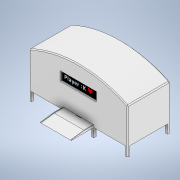
# Autodesk Inventor part: Twist Body
Saved by Autodesk Inventor 2021 (Build 250183000, 183)
## iProperties
Created: 2021-03-24
Part Number: Twist Body
Material: Generic
Document SubType Name: Modeling
Designer: calst
Density: 1 g/cm^3
Appearance: Smooth - White
Author: calst
Autodesk Inventor part; units mm, degrees
ref_plane "YZ Plane" through (0, 0, 0) normal (1, 0, 0) x (0, 1, 0)
ref_plane "XZ Plane" through (0, 0, 0) normal (0, 1, 0) x (-1, 0, 0)
ref_plane "XY Plane" through (0, 0, 0) normal (0, 0, 1) x (1, 0, 0)
sketch "Sketch1" plane through (0, 0, 0) normal (0, 1, 0) x (-1, 0, 0)
  line L0 (0, 0) -> (68.5, 0)
  line L1 (68.5, 0) -> (68.5, -94)
  line L2 (68.5, -94) -> (0, -94)
  line L3 (0, -94) -> (0, 0)
  dimension "d0" = 94
  dimension "d1" = 68.5
  constraints: 8 end point, 2 parallel, 1 horizontal, 1 perpendicular
  measures "d0" distance of L0.end L1.end
  measures "d1" distance of L1.end L2.end
extrude "Extrusion1" add sketch "Sketch1" along normal blind 4
sketch "Sketch2" plane through (0, 4, 0) normal (0, 1, 0) x (1, 0, 0)
  line L0 (0, 94) -> (-68.5, 94) projected
  line L1 (-68.5, 0) -> (0, 0) projected
  line L2 (-34.25, 0) -> (-39.25, 0)
  line L3 (-39.25, 0) -> (-39.25, 94)
  line L4 (-39.25, 94) -> (-29.25, 94)
  line L5 (-29.25, 94) -> (-29.25, 0)
  line L6 (-29.25, 0) -> (-34.25, 0)
  point P0 (-29.25, 0)
  dimension "d4" = 5
  dimension "d5" = 10
  constraints: 10 end point, 4 perpendicular, 1 midpoint, 1 point on line
  measures "d4" distance of L2.start L2.end
  measures "d5" distance of L3.end L4.end
extrude "Extrusion2" cut sketch "Sketch2" against normal blind 5
sketch "Sketch3" plane through (0, 4, 0) normal (0, 1, 0) x (1, 0, 0)
  line L0 (-39.25, 94) -> (-68.5, 94) projected
  line L1 (-68.5, 94) -> (-64.1699, 94)
  line L2 (-66, 89) -> (-68.5, 89)
  line L3 (-68.5, 89) -> (-68.5, 94)
  line L4 (-66, 89) -> (-66, 91.5)
  line L5 (-66, 91.5) -> (-64.1699, 91.5)
  line L6 (-64.1699, 94) -> (-68.5, 94)
  line L7 (-68.5, 94) -> (-68.5, 0) projected
  line L8 (-68.5, 89) -> (-68.5, 94)
  line L9 (0, 94) -> (-5, 94)
  line L10 (0, 94) -> (-29.25, 94) projected
  line L11 (-5, 91.5) -> (-2.5, 91.5)
  line L12 (-2.5, 91.5) -> (-2.5, 89)
  line L13 (0, 0) -> (0, 94) projected
  line L14 (0, 89) -> (0, 94)
  line L15 (-64.1699, 91.5) -> (-5, 91.5)
  line L16 (-64.1699, 94) -> (-5, 94)
  line L17 (0, 89) -> (0, 0)
  line L18 (0, 0) -> (-68.5, 0)
  line L19 (-68.5, 0) -> (-68.5, 89)
  line L20 (-66, 89) -> (-66, 2.5)
  line L21 (-68.5, 0) -> (-39.25, 0) projected
  line L22 (-66, 2.5) -> (-2.5, 2.5)
  line L23 (-2.5, 2.5) -> (-2.5, 89)
  dimension "d8" = 5
  dimension "d9" = 5
  dimension "d11" = 2.5
  dimension "d12" = 2.5
  dimension "d13" = 2.5
  dimension "d15" = 86.5
  constraints: 38 end point, 5 perpendicular, 4 collinear, 2 horizontal, 2 parallel, 1 point on line, 1 vertical
  measures "d8" distance of L5.end L2.end
  measures "d9" distance of L2.end L0.end
  measures "d11" distance of L9.end L11.start
  measures "d12" distance of L1.end L5.end
  measures "d13" distance of L2.start L4.end
  measures "d15" distance of L2.start L20.end
extrude "Extrusion3" add sketch "Sketch3" along normal blind 5
sketch "Sketch4" plane through (-29.25, 0, 0) normal (0, 0, 1) x (1, 0, 0)
  line L0 (-10, 4) -> (-36.75, 4) projected
  line L1 (26.75, 4) -> (0, 4) projected
  line L2 (-36.75, 4) -> (26.75, 4)
  line L3 (26.75, 4) -> (26.75, 5.1)
  line L4 (-36.75, 4) -> (-36.75, 5.1)
  line L5 (-36.75, 5.1) -> (26.75, 5.1)
  point P0 (29.25, 0)
  point P1 (-39.25, 9)
  dimension "d19" = 1.1
  dimension "d20" = 1.1
  constraints: 8 end point, 2 perpendicular, 1 collinear
  measures "d19" distance of L1.start L3.end
  measures "d20" distance of L0.end L4.end
extrude "Extrusion4" cut sketch "Sketch4" against normal blind 5
sketch "Sketch5" plane through (0, 9, 0) normal (0, 1, 0) x (1, 0, 0)
  line L0 (-66, 2.5) -> (-66, 91.5) projected
  line L1 (-68.5, 94) -> (-68.5, 0) projected
  line L2 (-66, 91.5) -> (-68.5, 91.5)
  line L3 (-68.5, 91.5) -> (-68.5, 94)
  line L4 (-68.5, 94) -> (-66, 94)
  line L5 (-66, 94) -> (-66, 91.5)
  line L6 (0, 0) -> (0, 94) projected
  line L7 (-2.5, 91.5) -> (-29.25, 91.5) projected
  line L8 (0, 94) -> (-2.5, 94)
  line L9 (-2.5, 94) -> (-2.5, 91.5)
  line L10 (-2.5, 91.5) -> (0, 91.5)
  line L11 (0, 91.5) -> (0, 94)
  line L12 (-68.5, 0.034) -> (-66, 0.034)
  line L13 (-66, 0.034) -> (-66, 2.534)
  line L14 (-66, 2.534) -> (-68.5, 2.534)
  line L15 (-68.5, 2.534) -> (-68.5, 0.034)
  line L16 (-2.5, 2.5) -> (-66, 2.5) projected
  line L17 (-68.5, 0) -> (0, 0) projected
  line L18 (-2.5, 2.5) -> (0, 2.5)
  line L19 (0, 2.5) -> (0, 0)
  line L20 (0, 0) -> (-2.5, 0)
  line L21 (-2.5, 0) -> (-2.5, 2.5)
  dimension "d23" = 2.5
  constraints: 32 end point, 8 parallel, 4 horizontal, 4 perpendicular, 2 point on line, 1 other
  measures "d23" distance of L12.end L13.end
extrude "Extrusion5" add sketch "Sketch5" along normal blind 30 contours L13 L12 L1 L14 L0 | L18 L6 L17 L21 | L2 L1 L4 L5 | L10 L9 L8 L6
sketch "Sketch6" plane through (0, 4, 0) normal (0, 1, 0) x (1, 0, 0)
  line L0 (-39.25, 94) -> (-68.5, 94) projected
  line L1 (-68.5, 94) -> (-66.2, 94)
  line L2 (-66.2, 94) -> (-66.2, 91.7)
  line L3 (-68.5, 91.5) -> (-66, 91.5) projected
  line L4 (0, 0) -> (0, 94) projected
  line L5 (0, 0) -> (-2.3, 0)
  line L6 (-29.25, 0) -> (0, 0) projected
  line L7 (-2.3, 0) -> (-2.3, 2.3)
  line L8 (-66.2, 91.7) -> (-2.3, 91.7)
  line L9 (-2.3, 91.7) -> (-2.3, 2.3)
  line L10 (-2.3, 2.3) -> (-66.2, 2.3)
  line L11 (-66.2, 2.3) -> (-66.2, 91.7)
  dimension "d26" = 2.3
  dimension "d27" = 2.3
  dimension "d28" = 2.3
  dimension "d29" = 2.3
  constraints: 16 end point, 3 perpendicular, 2 parallel, 2 point on line, 1 horizontal
  measures "d26" distance of L0.end L1.end
  measures "d27" distance of L1.end L2.end
  measures "d28" distance of L4.start L5.end
  measures "d29" distance of L5.end L7.end
extrude "Extrusion6" cut sketch "Sketch6" along normal blind 50
sketch "Sketch8" plane through (0, 0, 0) normal (1, 0, 0) x (0, 0, -1)
  line L0 (0, 4) -> (91.7, 4) projected
  line L1 (0, 4) -> (-20, 4)
  line L2 (-50, 0) -> (-20, 4)
  line L3 (0, 4) -> (0, 0) projected
  line L4 (-50, 0) -> (0, 0)
  dimension "d32" = 20
  constraints: 6 end point, 1 collinear, 1 horizontal
  measures "d32" distance of L0.start L1.end
extrude "Extrusion7" add sketch "Sketch8" against normal blind 68.5
sketch "Sketch10" plane through (0, 0, -94) normal (1, 0, 0) x (0, 0, -1)
  line L0 (-114, 4) -> (-94, 4) projected
  line L1 (-94, 5.1) -> (-91.7, 5.1) projected
  line L2 (-114, 5.1) -> (-94, 5.1)
  line L3 (-114, 4) -> (-144, 0) projected
  line L4 (-144, 0) -> (-144, 1.1)
  line L5 (-144, 1.1) -> (-114, 5.1)
  line L6 (-144, 0) -> (-114, 4)
  line L7 (-94, 4) -> (-94, 5.1)
  line L8 (-94, 4) -> (-91.7, 4) projected
  line L9 (-94, 4) -> (-114, 4)
  point P0 (-94, 0)
  dimension "d37" = 1.1
  constraints: 12 end point, 1 collinear, 1 perpendicular, 1 vertical
  measures "d37" distance of L3.end L4.end
extrude "Extrusion8" add sketch "Sketch10" against normal blind 1
sketch "Sketch11" plane through (-68.5, 4, 0) normal (-1, 0, 0) x (0, 0, 1)
  line L0 (50, -4) -> (20, 0) projected
  line L1 (50, -4) -> (50, -2.9) projected
  line L2 (50, -4) -> (50, -2.9)
  line L3 (20, 1.1) -> (0, 1.1) projected
  line L4 (50, -2.9) -> (20, 1.1)
  line L5 (20, 1.1) -> (0, 1.1)
  line L6 (0, 1.1) -> (0, 0) projected
  line L7 (0, 1.1) -> (0, 0)
  line L8 (20, 0) -> (0, 0) projected
  line L9 (0, 0) -> (20, 0)
  line L10 (50, -4) -> (-94, -4) projected
  line L11 (20, 0) -> (50, -4)
  point P0 (0, -4)
  constraints: 12 end point, 4 equal length, 1 perpendicular
extrude "Extrusion9" add sketch "Sketch11" against normal blind 1
sketch "Sketch15" plane through (-66.2, 4, -91.7) normal (0, 0, 1) x (1, 0, 0)
  line L0 (26.95, 0) -> (36.95, 0)
  line L1 (36.95, 0) -> (36.95, 1.1)
  line L2 (36.95, 1.1) -> (26.95, 1.1)
  line L3 (26.95, 1.1) -> (26.95, 0)
  point P0 (66.2, -4)
  dimension "d56" = 1.1
  constraints: 8 end point, 2 parallel, 1 horizontal, 1 perpendicular
  measures "d56" distance of L0.end L1.end
extrude "Extrusion13" cut sketch "Sketch15" against normal blind 94
sketch "Sketch17" plane through (0, 0, 0) normal (0, -1, 0) x (1, 0, 0)
  line L0 (-29.25, -81.7) -> (-24.25, -81.7)
  line L1 (-24.25, -81.7) -> (-24.25, -101.7)
  line L2 (-24.25, -101.7) -> (-29.25, -101.7)
  line L3 (-29.25, -101.7) -> (-29.25, -81.7)
  line L4 (-66, -2.3) -> (-2.5, -2.3) projected
  line L5 (-29.25, 0) -> (-39.25, 0) projected
  line L6 (-2.5, -2.3) -> (-66, -2.3) projected
  line L7 (-29.25, -2.3) -> (-29.25, -12.3)
  line L8 (-29.25, -91.7) -> (-29.25, 0) projected
  line L9 (-29.25, -12.3) -> (-24.25, -12.3)
  line L10 (-24.25, -12.3) -> (-24.25, 7.7)
  line L11 (-24.25, 7.7) -> (-29.25, 7.7)
  line L12 (-29.25, 7.7) -> (-29.25, -2.3)
  line L13 (-39.25, -2.3) -> (-39.25, -12.3)
  line L14 (-39.25, 0) -> (-39.25, -91.7) projected
  line L15 (-39.25, -12.3) -> (-44.25, -12.3)
  line L16 (-44.25, -12.3) -> (-44.25, 7.7)
  line L17 (-44.25, 7.7) -> (-39.25, 7.7)
  line L18 (-39.25, 7.7) -> (-39.25, -2.3)
  point P0 (0, 0)
  point P1 (-39.25, -81.7)
  dimension "d76" = 2.3
  dimension "d77" = 10
  dimension "d78" = 5
  dimension "d79" = 20
  constraints: 28 end point, 7 perpendicular, 6 point on line, 2 collinear, 1 horizontal
  measures "d76" distance between parallel lines of L4 L5
  measures "d77" distance of L7.start L7.end
  measures "d78" distance of L7.end L9.end
  measures "d79" distance of L9.end L10.end
extrude "Extrusion14" add sketch "Sketch17" along normal blind 20 contours L0 L1 L2 L3 | L13 L15 L16 L4 | L4 L16 L17 L18 L14 | L8 L12 L11 L10 L4 | L4 L10 L9 L7
fillet "Fillet1" radius 10 6 edges at (-26.75, -20, -81.7) (-26.75, -20, -101.7) (-26.75, -20, 7.7) (-26.75, -20, -12.3) (-41.75, -20, -12.3) (-41.75, -20, 7.7)
sketch "Sketch19" plane through (-24.25, 0, 7.7) normal (1, 0, 0) x (0, 0, -1)
  arc A0 (0, -10) -> (20, -10) centre (10, -10) ccw projected
  circle A1 centre (10, -10) radius 2.5
  arc A2 (89.4, -10) -> (109.4, -10) centre (99.4, -10) ccw projected
  circle A3 centre (99.4, -10) radius 2.5
  point P0 (7.7, 0)
  dimension "d80" = 5
  dimension "d81" = 5
  constraints: 2 centre point, 2 coincident
  measures "d80" diameter of A1
  measures "d81" diameter of A3
extrude "Extrusion16" cut sketch "Sketch19" against normal blind 30
sketch "Sketch21" plane through (0, 0, 0) normal (0, -1, 0) x (1, 0, 0)
  line L0 (-68.5, -94) -> (-63.5, -94)
  line L1 (-63.5, -94) -> (-63.5, -89)
  line L2 (-63.5, -89) -> (-68.5, -89)
  line L3 (-68.5, -89) -> (-68.5, -94)
  line L4 (-67.5, 50) -> (-68.5, 50) projected
  line L5 (0, 50) -> (-1, 50) projected
  line L6 (0, -94) -> (-2.5, -94) projected
  line L7 (0, -94) -> (-5, -94)
  line L8 (-5, -94) -> (-5, -89)
  line L9 (-5, -89) -> (0, -89)
  line L10 (0, -89) -> (0, -94)
  dimension "d84" = 5
  dimension "d85" = 5
  constraints: 16 end point, 4 parallel, 2 horizontal, 2 perpendicular
  measures "d84" distance of L0.end L1.end
  measures "d85" distance of L1.end L2.end
extrude "Extrusion17" add sketch "Sketch21" along normal blind 20
sketch "Sketch23" plane through (0, 9, -91.5) normal (1, 0, 0) x (0, 0, -1)
  point P0 (-91.5, -9)
sketch "Sketch24" plane through (0, 0, 0) normal (0, -1, 0) x (1, 0, 0)
  line L0 (0, 0) -> (-5, 0)
  line L1 (-5, 0) -> (-5, -5)
  line L2 (-5, -5) -> (0, -5)
  line L3 (0, -5) -> (0, 0)
  line L4 (-68.5, -0.034) -> (-68.5, 0) projected
  line L5 (-68.5, 0) -> (-63.5, 0)
  line L6 (-63.5, 0) -> (-63.5, -5)
  line L7 (-63.5, -5) -> (-68.5, -5)
  line L8 (-68.5, -5) -> (-68.5, 0)
  dimension "d94" = 5
  dimension "d95" = 5
  dimension "d96" = 5
  constraints: 16 end point, 4 parallel, 2 horizontal, 2 perpendicular
  measures "d94" distance of L2.end L1.end
  measures "d95" distance of L0.end L1.end
  measures "d96" distance of L6.end L7.end
extrude "Extrusion18" add sketch "Sketch24" along normal blind 20
sketch "Sketch25" plane through (0, 9, -91.5) normal (1, 0, 0) x (0, 0, -1)
  line L0 (-91.466, 0) -> (-91.5, 0) projected
  line L1 (-9.8, -9) -> (2.5, -9) projected
  line L2 (-91.5, 0) -> (2.5, 0)
  line L3 (2.5, 0) -> (2.5, -9)
  line L4 (2.5, -9) -> (-91.5, -9)
  line L5 (-91.5, -9) -> (-91.5, 0)
  point P0 (-91.5, -9)
  constraints: 8 end point, 2 parallel, 1 horizontal, 1 perpendicular
extrude "Extrusion19" add sketch "Sketch25" along normal blind 75
sketch "Sketch26" plane through (-68.5, 9, -0.034) normal (-1, 0, 0) x (0, 0, 1)
  line L0 (0.034, -9) -> (0.034, -29) projected
  line L1 (-93.966, 0) -> (0.034, 0)
  line L2 (0.034, 0) -> (0.034, -9)
  line L3 (0.034, -9) -> (-93.966, -9)
  line L4 (-93.966, -9) -> (-93.966, 0)
  constraints: 8 end point, 2 parallel, 1 horizontal, 1 perpendicular
extrude "Extrusion20" add sketch "Sketch26" along normal blind 75
sketch "Sketch28" plane through (0, 0, 0) normal (0, -1, 0) x (1, 0, 0)
  line L0 (-68.5, -94) -> (-143.5, -94) projected
  line L1 (-143.5, -94) -> (-138.5, -94)
  line L2 (-138.5, -94) -> (-138.5, -89)
  line L3 (-138.5, -89) -> (-143.5, -89)
  line L4 (-143.5, -89) -> (-143.5, -94)
  line L5 (-143.5, -94) -> (-143.5, 0) projected
  line L6 (-143.5, 0) -> (-138.5, 0)
  line L7 (-138.5, 0) -> (-138.5, -5)
  line L8 (-138.5, -5) -> (-143.5, -5)
  line L9 (-143.5, -5) -> (-143.5, 0)
  line L10 (0, -94) -> (75, -94) projected
  line L11 (75, -94) -> (70, -94)
  line L12 (70, -94) -> (70, -89)
  line L13 (70, -89) -> (75, -89)
  line L14 (75, -89) -> (75, -94)
  line L15 (75, -94) -> (75, 0) projected
  line L16 (75, 0) -> (70, 0)
  line L17 (70, 0) -> (70, -5)
  line L18 (70, -5) -> (75, -5)
  line L19 (75, -5) -> (75, 0)
  point P0 (0, 0)
  dimension "d103" = 5
  dimension "d104" = 5
  dimension "d105" = 5
  dimension "d106" = 5
  dimension "d107" = 5
  dimension "d108" = 5
  constraints: 32 end point, 8 parallel, 4 horizontal, 4 perpendicular, 2 point on line
  measures "d103" distance of L3.end L2.end
  measures "d104" distance of L12.end L13.end
  measures "d105" distance of L18.end L17.end
  measures "d106" distance of L6.end L7.end
  measures "d107" distance of L1.end L2.end
  measures "d108" distance of L16.end L17.end
extrude "Extrusion21" add sketch "Sketch28" along normal blind 20
sketch "Sketch29" plane through (0, 9, 0) normal (0, 1, 0) x (1, 0, 0)
  point P0 (0, 0)
sketch "Sketch30" plane through (0, 9, 0) normal (0, 1, 0) x (1, 0, 0)
  line L0 (2.7, 89) -> (70, 89)
  line L1 (70, 89) -> (70, 5)
  line L2 (70, 5) -> (2.7, 5)
  line L3 (2.7, 5) -> (2.7, 89)
  line L4 (-138.5, 94) -> (-138.5, 89) projected
  line L5 (-138.5, 89) -> (-71.2, 89)
  line L6 (-71.2, 89) -> (-71.2, 5)
  line L7 (-71.2, 5) -> (-138.5, 5)
  line L8 (-138.5, 5) -> (-138.5, 89)
  line L9 (-2.5, 0) -> (-143.5, 0) projected
  line L10 (-66.2, 2.534) -> (-66.2, 91.5) projected
  line L11 (0, 94) -> (75, 94) projected
  line L12 (75, 94) -> (75, 0) projected
  line L13 (-2.3, 91.5) -> (-2.3, 2.5) projected
  point P0 (0, 0)
  dimension "d111" = 5
  dimension "d112" = 5
  dimension "d113" = 5
  dimension "d114" = 5
  dimension "d115" = 5
  constraints: 16 end point, 4 parallel, 2 horizontal, 2 perpendicular, 1 point on line
  measures "d111" distance between parallel lines of L9 L7
  measures "d112" distance between parallel lines of L10 L6
  measures "d113" distance between parallel lines of L11 L0
  measures "d114" distance between parallel lines of L12 L1
  measures "d115" distance between parallel lines of L13 L3
extrude "Extrusion22" cut sketch "Sketch30" against normal blind 5
sketch "Sketch32" plane through (0, 9, 0) normal (0, 1, 0) x (1, 0, 0)
  line L0 (-68.5, 94) -> (-143.5, 94) projected
  line L1 (75, 5) -> (75, 0) projected
  line L2 (-143.5, 94) -> (75, 94)
  line L3 (75, 94) -> (75, 0)
  line L4 (75, 0) -> (-143.5, 0)
  line L5 (-143.5, 0) -> (-143.5, 94)
  line L6 (-71.2, 89) -> (-71.2, 5) projected
  line L7 (-138.5, 89) -> (-71.2, 89)
  line L8 (-71.2, 89) -> (-71.2, 5)
  line L9 (-71.2, 5) -> (-138.5, 5)
  line L10 (-138.5, 5) -> (-138.5, 89)
  line L11 (70, 89) -> (70, 5) projected
  line L12 (2.7, 89) -> (70, 89)
  line L13 (70, 89) -> (70, 5)
  line L14 (70, 5) -> (2.7, 5)
  line L15 (2.7, 5) -> (2.7, 89)
  line L16 (-66.2, 2.534) -> (-66.2, 91.5) projected
  line L17 (-2.5, 91.7) -> (-2.3, 91.7) projected
  line L18 (-66.2, 2.534) -> (-2.3, 2.534)
  line L19 (-2.3, 2.534) -> (-2.3, 91.7)
  line L20 (-2.3, 91.7) -> (-66.2, 91.7)
  line L21 (-66.2, 91.7) -> (-66.2, 2.534)
  point P0 (0, 0)
  constraints: 32 end point, 8 parallel, 4 horizontal, 4 perpendicular
extrude "Extrusion23" add sketch "Sketch32" along normal blind 30
chamfer "Chamfer1" distance 2 angle 45 2 edges at (-143.5, 9.5, 0) (75, 9.5, 0)
sketch "Sketch34" plane through (-138.5, 39, -5) normal (1, 0, 0) x (0, 0, -1)
  line L0 (-3, 0) -> (-3, -59) projected
  line L1 (0, 0) -> (84, 0) projected
  line L2 (-3, 0) -> (84, 0)
  line L3 (84, 0) -> (84, -2.5)
  line L4 (84, 0) -> (84, -35) projected
  line L5 (84, -2.5) -> (-3, -2.5)
  line L6 (-3, -2.5) -> (-3, 0)
  point P0 (-5, -39)
  point P1 (84, -15)
  point P2 (-3, -2.5)
  dimension "d129" = 2.5
  constraints: 8 end point, 2 perpendicular, 1 collinear, 1 point on line
  measures "d129" distance of L1.end L3.end
extrude "Extrusion25" add sketch "Sketch34" along normal blind 68
sketch "Sketch35" plane through (2.7, 39, -5) normal (1, 0, 0) x (0, 0, -1)
  line L0 (0, -2.5) -> (0, -35) projected
  line L1 (0, 0) -> (0, -2.5)
  line L2 (84, -2.5) -> (84, -35) projected
  line L3 (0, -2.5) -> (84, -2.5)
  line L4 (84, -2.5) -> (84, 0)
  line L5 (84, 0) -> (0, 0)
  point P0 (-5, -39)
  point P1 (0, -15)
  point P2 (84, -15)
  constraints: 8 end point, 2 perpendicular, 1 parallel, 1 vertical
extrude "Extrusion26" add sketch "Sketch35" along normal blind 68
sketch "Sketch36" plane through (0, 39, 0) normal (0, 1, 0) x (1, 0, 0)
  line L0 (-66.2, 2.534) -> (-66.2, 91.7) projected
  line L1 (-143.5, 94) -> (-143.5, 2) projected
  line L2 (-68.5, 0) -> (-138.5, 0) projected
  line L3 (-94.85, 42.117) -> (-114.85, 42.117)
  line L4 (-114.85, 42.117) -> (-114.85, 52.117)
  line L5 (-114.85, 52.117) -> (-94.85, 52.117)
  line L6 (-94.85, 52.117) -> (-94.85, 42.117)
  line L7 (-94.85, 42.117) -> (-114.85, 52.117) construction
  line L8 (-114.85, 42.117) -> (-94.85, 52.117) construction
  line L9 (46.35, 42.117) -> (26.35, 42.117)
  line L10 (26.35, 42.117) -> (26.35, 52.117)
  line L11 (26.35, 52.117) -> (46.35, 52.117)
  line L12 (46.35, 52.117) -> (46.35, 42.117)
  line L13 (46.35, 42.117) -> (26.35, 52.117) construction
  line L14 (26.35, 42.117) -> (46.35, 52.117) construction
  line L15 (-141.5, 0) -> (73, 0) projected
  line L16 (75, 2) -> (75, 94) projected
  point P0 (0, 0)
  point P1 (36.35, 47.117)
  dimension "d134" = 20
  dimension "d135" = 10
  dimension "d136" = 42.117
  dimension "d137" = 28.65
  dimension "d138" = 20
  dimension "d139" = 42.117
  dimension "d140" = 28.65
  constraints: 24 end point, 4 parallel, 2 horizontal, 2 midpoint, 2 perpendicular
  measures "d134" distance of L4.end L5.end
  measures "d135" distance of L3.end L4.end
  measures "d136" distance between parallel lines of L2 L3
  measures "d137" distance between parallel lines of L1 L4
  measures "d138" distance of L10.end L11.end
  measures "d139" distance between parallel lines of L15 L9
  measures "d140" distance between parallel lines of L16 L12
extrude "Extrusion27" cut sketch "Sketch36" against normal blind 2.5
sketch "Sketch37" plane through (-138.5, 36.5, -89) normal (0, -1, 0) x (1, 0, 0)
  line L0 (23.65, 46.883) -> (43.65, 46.883) projected
  line L1 (23.65, 46.883) -> (43.65, 46.883)
  line L2 (43.65, 46.883) -> (43.65, 51.883)
  line L3 (43.65, 51.883) -> (23.65, 51.883)
  line L4 (23.65, 51.883) -> (23.65, 46.883)
  line L5 (164.85, 46.883) -> (184.85, 46.883)
  line L6 (184.85, 46.883) -> (184.85, 51.883)
  line L7 (184.85, 51.883) -> (164.85, 51.883)
  line L8 (164.85, 51.883) -> (164.85, 46.883)
  point P0 (138.5, 89)
  point P1 (43.65, 46.883)
  dimension "d143" = 5
  dimension "d144" = 20
  constraints: 16 end point, 4 parallel, 2 horizontal, 2 perpendicular
  measures "d143" distance of L3.end L0.start
  measures "d144" distance of L7.end L6.end
extrude "Extrusion28" add sketch "Sketch37" along normal blind 20
fillet "Fillet2" radius 10 4 edges at (46.35, 16.5, -39.617) (26.35, 16.5, -39.617) (-94.85, 16.5, -39.617) (-114.85, 16.5, -39.617)
sketch "Sketch38" plane through (26.35, 36.5, -37.117) normal (0, 0, 1) x (1, 0, 0)
  arc A0 (0, -10) -> (20, -10) centre (10, -10) ccw projected
  circle A1 centre (10, -10) radius 2.5
  arc A2 (-141.2, -10) -> (-121.2, -10) centre (-131.2, -10) ccw projected
  circle A3 centre (-131.2, -10) radius 2.5
  point P0 (-26.35, -36.5)
  dimension "d148" = 5
  dimension "d149" = 5
  constraints: 2 centre point, 2 coincident
  measures "d148" diameter of A1
  measures "d149" diameter of A3
extrude "Extrusion29" cut sketch "Sketch38" against normal blind 5
sketch "Sketch39" plane through (0, 39, 0) normal (0, 1, 0) x (1, 0, 0)
  line L0 (-143.5, 94) -> (-143.5, 2) projected
  line L1 (75, 94) -> (-143.5, 94) projected
  line L2 (-141.5, 0) -> (73, 0) projected
  line L3 (75, 2) -> (75, 94) projected
  line L4 (75, 2) -> (73, 0) projected
  line L5 (-141.5, 0) -> (-143.5, 2) projected
  line L6 (-66.2, 91.7) -> (-2.3, 91.7) projected
  line L7 (-2.3, 2.534) -> (-66.2, 2.534) projected
  line L8 (-39.25, 91.7) -> (-66.2, 91.7) projected
  line L9 (-66.2, 91.7) -> (-141.2, 91.7)
  line L10 (-2.3, 91.7) -> (72.7, 91.7)
  line L11 (-66, 0) -> (-66, 2.3) projected
  line L12 (-66, 2.3) -> (-141.2, 2.3)
  line L13 (-141.2, 2.3) -> (-141.2, 91.7)
  line L14 (-66, 2.3) -> (-2.5, 2.3) projected
  line L15 (-66, 2.3) -> (72.7, 2.3)
  line L16 (72.7, 91.7) -> (72.7, 2.3)
  line L17 (-66.2, 91.7) -> (-2.3, 91.7)
  line L18 (-2.5, 2.3) -> (-66, 2.3)
  line L19 (-143.5, 94) -> (75, 94)
  line L20 (75, 2) -> (75, 94)
  line L21 (73, 0) -> (75, 2)
  line L22 (75, 2) -> (73, 0)
  line L23 (73, 0) -> (70, 0) projected
  line L24 (-141.5, 0) -> (73, 0)
  line L25 (-143.5, 89) -> (-143.5, 94) projected
  line L26 (-143.5, 2) -> (-143.5, 94)
  line L27 (-141.5, 0) -> (-143.5, 2)
  point P0 (0, 0)
  dimension "d153" = 2.3
  dimension "d154" = 2.3
  dimension "d155" = 2.3
  constraints: 30 end point, 4 horizontal, 2 collinear, 2 perpendicular, 2 vertical, 1 parallel, 1 point on line
  measures "d153" distance between parallel lines of L1 L9
  measures "d154" distance from line of L0 L9.end
  measures "d155" distance from line of L3 L10.end
extrude "Extrusion30" add sketch "Sketch39" along normal blind 40
sketch "Sketch40" plane through (-29.25, 5.1, -94) normal (0, 0, -1) x (-1, 0, 0)
  line L0 (114.25, 73.9) -> (112.25, 73.9) projected
  arc A0 (114.25, 73.9) -> (-104.25, 73.9) centre (5, -150.9654) ccw
  line L1 (-104.25, 73.9) -> (114.25, 73.9)
  line L2 (-102.25, 73.9) -> (-102.25, -25.1) projected
  point P0 (-29.25, -5.1)
  dimension "d158" = 250
  constraints: 2 end point, 2 point on circle, 1 centre point, 1 perpendicular
  measures "d158" radius of A0
extrude "Extrusion31" add sketch "Sketch40" against normal blind 94
chamfer "Chamfer2" distance 2 angle 45 1 edges at (-34.25, 104.1346, 0)
chamfer "Chamfer3" distance 2 angle 45 5 edges at (-143.5, 29.5, -94) (75, 29.5, -94) (-34.25, 104.1346, -94) (-143.5, 79, -48) (75, 79, -48)
sketch "Sketch41" plane through (-66, 5.1, 0) normal (0, 0, 1) x (1, 0, 0)
  arc A0 (139, 72.6446) -> (-75.5, 72.6446) centre (31.75, -150.9654) ccw projected
  line L0 (31.75, 47.0346) -> (71.75, 47.0346)
  line L1 (71.75, 47.0346) -> (71.75, 67.0346)
  line L2 (31.75, 47.0346) -> (-8.25, 47.0346)
  line L3 (-8.25, 47.0346) -> (-8.25, 67.0346)
  line L4 (-8.25, 67.0346) -> (71.75, 67.0346)
  point P0 (66, -5.1)
  dimension "d170" = 40
  dimension "d171" = 20
  dimension "d172" = 40
  dimension "d173" = 20
  constraints: 10 end point, 2 perpendicular, 1 horizontal
  measures "d170" distance of L0.start L0.end
  measures "d171" distance of L0.end L1.end
  measures "d172" distance of L0.start L2.end
  measures "d173" distance of L2.end L3.end
extrude "Extrusion32" cut sketch "Sketch41" against normal blind 2.2
ref_plane "Work Plane1" through (-66, 5.1, 28.05) normal (0, 0, 1) x (1, 0, 0)
sketch "Sketch43" plane through (-66, 5.1, 28.05) normal (0, 0, 1) x (1, 0, 0)
  line L0 (-6.2731, 67.1185) -> (70.6599, 67.1185) construction
  line L1 (70.6599, 67.1185) -> (70.6599, 47.1186) construction
  line L2 (70.6599, 47.1186) -> (-6.2731, 47.1186) construction
  line L3 (-6.2731, 47.1186) -> (-6.2731, 67.1185) construction
  point P0 (66, -5.1)
  constraints: 2 other
decal "Decal1"
body "Solid1"
